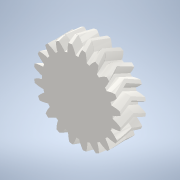
# Autodesk Inventor part: Spur Gear1
Saved by Autodesk Inventor 2021 (Build 250183000, 183)
## iProperties
Created: 2021-06-27
Part Number: Spur Gear1
Material: Steel
Document SubType Name: Modeling
Designer: Łukasz
Categories: <?xml version="1.0" encoding="UTF-16"?> <MemberInstance><Categories><FamilyTemplate><FamilyTemplateParameter ValueType="xs:double" Id="1" ObjectReferenceKey="da_z" ObjectType="kUserParameterObject"/><FamilyTemplateParameter ValueType="xs:double" Id="2" ObjectReferenceKey="da_b" ObjectType="kUserParameterObject"/><FamilyTemplateParameter ValueType="xs:double" Id="3" ObjectReferenceKey="da_beta" ObjectType="kUserParameterObject"/><FamilyTemplateParameter ValueType="xs:double" Id="4" ObjectReferenceKey="da_da" ObjectType="kUserParameterObject"/><FamilyTemplateParameter ValueType="xs:double" Id="5" ObjectReferenceKey="da_aw" ObjectType="kUserParameterObject"/><FamilyTemplateParameter ValueType="xs:string" Id="6" ObjectReferenceKey="EAIAABAAAACIAQAAAAAAAIAAAAAAAAAA" ObjectType="83910656" SubObjectId="SurfaceGeometry"/></FamilyTemplate><ParamToTemplateMap><ParamToTemplate CategoryParameter="//CategoryParameter[@InternalName='046C89C9-8512-4d59-83FE-43B91F4F132A']" TemplateParameter="1"/><ParamToTemplate CategoryParameter="//CategoryParameter[@InternalName='2552DF32-E462-4b46-AEBF-C6C7768E72AC']" TemplateParameter="2"/><ParamToTemplate CategoryParameter="//CategoryParameter[@InternalName='C9EE641D-15FC-4fae-A226-E94C4372FDD7']" TemplateParameter="3"/><ParamToTemplate><ParamToTemplate CategoryParameter="//CategoryParameter[@InternalName='00B6519A-459B-49c7-AD84-2E56D39A5744']" ConstantValue="0.022987"/></ParamToTemplate><ParamToTemplate><ParamToTemplate CategoryParameter="//CategoryParameter[@InternalName='04B31F0E-C7A6-4894-AA32-9629BEFACF47']" ConstantValue="1.000000"/></ParamToTemplate><ParamToTemplate><ParamToTemplate CategoryParameter="//CategoryParameter[@InternalName='43CBEC2E-7847-49e7-A936-2F7889FCB2D9']" ConstantValue="0.250000"/></ParamToTemplate><ParamToTemplate><ParamToTemplate CategoryParameter="//CategoryParameter[@InternalName='B1EFC894-105D-4ebd-86BF-FA20ED196853']" ConstantValue="0.350000"/></ParamToTemplate><ParamToTemplate><ParamToTemplate CategoryParameter="//CategoryParameter[@InternalName='51175063-3D10-4879-93E8-6246FE8B403D']" ConstantValue="2060000000.000000"/></ParamToTemplate><ParamToTemplate><ParamToTemplate CategoryParameter="//CategoryParameter[@InternalName='A3A52E27-4454-46a9-B0BD-C932399B70AF']" ConstantValue="0.300000"/></ParamToTemplate><ParamToTemplate><ParamToTemplate CategoryParameter="//CategoryParameter[@InternalName='91B76062-C214-41d9-B1B9-14D2AB99603D']" ConstantValue="0.200000"/></ParamToTemplate><ParamToTemplate><ParamToTemplate CategoryParameter="//CategoryParameter[@InternalName='374E806E-8B8A-4dda-A9AA-1039D6500AD2']" ConstantValue="5.000000"/></ParamToTemplate><ParamToTemplate><ParamToTemplate CategoryParameter="//CategoryParameter[@InternalName='2D373A89-B862-43d6-8D0B-0CBF12AB9F6C']" ConstantValue="0.349066"/></ParamToTemplate><ParamToTemplate CategoryParameter="//CategoryParameter[@InternalName='37777632-D6A2-4fac-9D53-DB8ACD95C989']" TemplateParameter="4"/><ParamToTemplate CategoryParameter="//CategoryParameter[@InternalName='FD1017F1-B727-4f7e-9707-0F86F1FF9423']" TemplateParameter="5"/><ParamToTemplate><ParamToTemplate CategoryParameter="//CategoryParameter[@InternalName='9E1B4470-B2D3-4ff1-B813-535BB4CDF51A']" ConstantValue="9000000.000000"/></ParamToTemplate><ParamToTemplate><ParamToTemplate CategoryParameter="//CategoryParameter[@InternalName='F8452263-BFF6-458c-9FB1-07C4B99E95CD']" ConstantValue="11400000.000000"/></ParamToTemplate><ParamToTemplate><ParamToTemplate CategoryParameter="//CategoryParameter[@InternalName='3E3BB259-FD49-497f-8171-6EBC954A3479']" ConstantValue="2.000000"/></ParamToTemplate><ParamToTemplate CategoryParameter="//CategoryParameter[@InternalName='27C3BAF2-7550-4e4b-AE2C-0DB134B7D9B7']" TemplateParameter="6"/></ParamToTemplateMap><Category DisplayName="Gear" InternalName="DC85795E-93AB-48d5-8EEE-5A27447B64BD" Mnemonic="Gear"><CategoryParameter DisplayName="z" InternalName="046C89C9-8512-4d59-83FE-43B91F4F132A" Mnemonic="z"/><CategoryParameter DisplayName="b" InternalName="2552DF32-E462-4b46-AEBF-C6C7768E72AC" Mnemonic="b"/><CategoryParameter DisplayName="||b|" InternalName="C9EE641D-15FC-4fae-A226-E94C4372FDD7" Mnemonic="beta"/><CategoryParameter DisplayName="x" InternalName="00B6519A-459B-49c7-AD84-2E56D39A5744" Mnemonic="x"/><CategoryParameter DisplayName="a*" InternalName="04B31F0E-C7A6-4894-AA32-9629BEFACF47" Mnemonic="a"/><CategoryParameter DisplayName="c*" InternalName="43CBEC2E-7847-49e7-A936-2F7889FCB2D9" Mnemonic="c"/><CategoryParameter DisplayName="r|.f|*" InternalName="B1EFC894-105D-4ebd-86BF-FA20ED196853" Mnemonic="rf"/><CategoryParameter DisplayName="E" InternalName="51175063-3D10-4879-93E8-6246FE8B403D" Mnemonic="E"/><CategoryParameter DisplayName="||m|" InternalName="A3A52E27-4454-46a9-B0BD-C932399B70AF" Mnemonic="mi"/><Category DisplayName="SpurGear" InternalName="26C5A22E-A91E-4dfd-A3B3-23CCAFAE1764" Mnemonic="SpurGear"><CategoryParameter DisplayName="m" InternalName="91B76062-C214-41d9-B1B9-14D2AB99603D" Mnemonic="m"/><CategoryParameter DisplayName="P" InternalName="374E806E-8B8A-4dda-A9AA-1039D6500AD2" Mnemonic="PP"/><CategoryParameter DisplayName="||a|" InternalName="2D373A89-B862-43d6-8D0B-0CBF12AB9F6C" Mnemonic="alpha"/><CategoryParameter DisplayName="d|.a|" InternalName="37777632-D6A2-4fac-9D53-DB8ACD95C989" Mnemonic="da"/><CategoryParameter DisplayName="a|.w|" InternalName="FD1017F1-B727-4f7e-9707-0F86F1FF9423" Mnemonic="aw"/><CategoryParameter DisplayName="||s||.Flim|" InternalName="9E1B4470-B2D3-4ff1-B813-535BB4CDF51A" Mnemonic="sFlim"/><CategoryParameter DisplayName="||s||.Hlim|" InternalName="F8452263-BFF6-458c-9FB1-07C4B99E95CD" Mnemonic="sHlim"/><CategoryParameter DisplayName="type" InternalName="3E3BB259-FD49-497f-8171-6EBC954A3479" Mnemonic="type"/><CategoryParameter DisplayName="PitchDiameter" InternalName="27C3BAF2-7550-4e4b-AE2C-0DB134B7D9B7" Mnemonic="IDS_PITCHDIAM"/></Category></Category></Categories></MemberInstance>
Density: 1 g/cm^3
Appearance: Steel
CustomPartVersion: 1
Author: Łukasz
Autodesk Inventor part; units mm, degrees
ref_plane "YZ Plane" through (0, 0, 0) normal (1, 0, 0) x (0, 1, 0)
ref_plane "XZ Plane" through (0, 0, 0) normal (0, 1, 0) x (-1, 0, 0)
ref_plane "XY Plane" through (0, 0, 0) normal (0, 0, 1) x (1, 0, 0)
sketch "Sketch1" plane through (0, 0, 0) normal (0, 0, 1) x (1, 0, 0)
  circle A0 centre (0, 0) radius 25.1392
  dimension "d0" = 50.2784
  constraints: 1 centre point
  measures "d0" diameter of A0
extrude "Extrusion1" add sketch "Sketch1" along normal blind 7
ref_plane "Work Plane2" through (0, 0, 3.5) normal (0, 0, 1) x (1, 0, 0)
sketch "Sketch2" plane through (0, 0, 0) normal (0, 0, -1) x (-1, 0, 0)
  circle A0 centre (0, 0) radius 25.1392 projected
  circle A1 centre (0, 0) radius 23.094
  dimension "d3" = 46.188
  constraints: 1 centre point, 1 coincident
  measures "d3" diameter of A1
surface extrude "Pitch Diameter" sketch "Sketch2" against normal through all shown no curves A1
ref_plane "Work Plane8" through (0, 0, 0) normal (0.9876883, 0.1564345, 0) x (0, 0, 1)
ref_plane "Work Plane9" through (0, 0, 0) normal (1, 0, 0) x (0, 1, 0)
spur gear teeth "Spur Gear" teeth 20 pitch diameter 46.188 tip diameter 50.2784 root diameter 41.28 face width 7 helix angle 30 hand left start plane through (0, 0, 0) normal (0, 0, -1) x (-1, 0, 0)
sketch "Sketch4" plane through (0, 0, 7) normal (0, 0, 1) x (1, 0, 0)
  circle A0 centre (0, 0) radius 11
  dimension "d52" = 22
  constraints: 1 centre point, 1 coincident
  measures "d52" diameter of A0
extrude "Extrusion3" cut sketch "Sketch4" against normal up to surface (7 mm away)
mirror "Mirror2" about plane through (0, 0, 0) normal (0, 0, -1) bodies 1 separate body
equation "\"d0\" = da_da"
equation "\"d1\" = da_b"
equation "\"d3\" = da_d"
equation "\"d53\" = d52"
equation "\"d16\" = da_aw"
equation "\"d43\" = da_aw"
equation "\"d46\" = da_aw"
equation "\"da_da\" = 50.27844"
equation "\"da_b\" = 7"
equation "\"da_d\" = 46.188022"
equation "\"da_aw\" = 69.419188"
body "Solid1"
body "Srf1"
body "Solid3"
